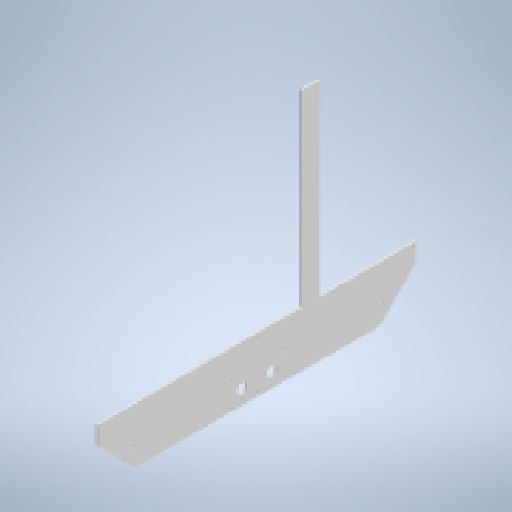
# Autodesk Inventor part: Outside Chassi Plate low
Saved by Autodesk Inventor 2023 (Build 270158000, 158)
## iProperties
Created: 2022-09-05
Part Number: Outside Chassi Plate low
Material: Generic
Document SubType Name: Modeling
Designer: deli
Density: 1 g/cm^3
Appearance: Default
Author: deli
Autodesk Inventor part; units mm, degrees
ref_plane "YZ Plane" through (0, 0, 0) normal (1, 0, 0) x (0, 1, 0)
ref_plane "XZ Plane" through (0, 0, 0) normal (0, 1, 0) x (-1, 0, 0)
ref_plane "XY Plane" through (0, 0, 0) normal (0, 0, 1) x (1, 0, 0)
sketch "Sketch1" plane through (0, 0, 0) normal (1, 0, 0) x (0, 1, 0)
  line L0 (-213.0456, 506.9498) -> (-238.0456, 506.9498)
  line L1 (-238.0456, 506.9498) -> (-289.5596, 456.0589)
  line L2 (-213.0456, 56.9498) -> (-238.0456, 56.9498)
  circle A0 centre (-263.0456, 456.9498) radius 2
  circle A1 centre (-263.0456, 456.9498) radius 48 construction
  arc A2 (-251.1195, 456.4491) -> (-274.9659, 457.5739) centre (-263.0456, 456.9498) ccw construction
  circle A3 centre (-263.0456, 106.9498) radius 48 construction
  arc A4 (-274.9659, 106.3258) -> (-251.1195, 107.4505) centre (-263.0456, 106.9498) ccw construction
  circle A5 centre (-263.0456, 106.9498) radius 2
  circle A6 centre (-270.2956, 303.2411) radius 7
  circle A7 centre (-270.2956, 260.6586) radius 7
  circle A8 centre (-270.2956, 303.2411) radius 18.75 construction
  circle A9 centre (-270.2956, 260.6586) radius 18.75 construction
  arc A10 (-283.0106, 303.9067) -> (-257.5745, 302.707) centre (-270.2956, 303.2411) ccw construction
  arc A11 (-257.5745, 261.1927) -> (-283.0106, 259.9929) centre (-270.2956, 260.6586) ccw construction
  line L3 (-251.1195, 456.4491) -> (-257.5745, 302.707) construction
  line L4 (-283.0106, 303.9067) -> (-274.9659, 457.5739) construction
  line L5 (-257.5745, 261.1927) -> (-251.1195, 107.4505) construction
  line L6 (-274.9659, 106.3258) -> (-283.0106, 259.9929) construction
  circle A12 centre (-255.8131, 281.9498) radius 2
  circle A13 centre (-284.7782, 281.9498) radius 2
  circle A14 centre (-286.0456, 320.3437) radius 2
  circle A15 centre (-286.0456, 243.5559) radius 2
  circle A16 centre (-252.9008, 245.2319) radius 2
  circle A17 centre (-218.0456, 501.9498) radius 2
  circle A18 centre (-218.0456, 61.9498) radius 2
  arc A19 (-291.0456, 229.9036) -> (-291.0456, 229.9036) centre (-268.2956, 229.9036) ccw
  line L7 (-291.0456, 189.1468) -> (-291.0456, 229.9036)
  arc A20 (-291.0456, 189.1468) -> (-291.0456, 189.1468) centre (-268.2956, 189.1468) ccw
  arc A21 (-289.5596, 456.0589) -> (-291.0456, 452.5019) centre (-286.0456, 452.5019) ccw
  line L8 (-291.0456, 452.5019) -> (-291.0456, 229.9036)
  line L9 (-238.0456, 56.9498) -> (-289.5596, 107.8407)
  line L10 (-291.0456, 189.1468) -> (-291.0456, 111.3977)
  circle A22 centre (-252.9008, 318.6677) radius 2
  arc A23 (-291.0456, 111.3977) -> (-289.5596, 107.8407) centre (-286.0456, 111.3977) ccw
  circle A24 centre (-218.0456, 391.9498) radius 2
  circle A25 centre (-218.0456, 281.9498) radius 2
  circle A26 centre (-218.0456, 171.9498) radius 2
  circle A27 centre (-286.0456, 359.8587) radius 2
  circle A28 centre (-286.0456, 399.3738) radius 2
  line L11 (51.9544, 193.3998) -> (-213.0456, 193.3998)
  line L12 (-213.0456, 218.7998) -> (51.9544, 218.7998)
  line L13 (51.9544, 218.7998) -> (51.9544, 193.3998)
  line L14 (-213.0456, 506.9498) -> (-213.0456, 218.7998)
  line L15 (-213.0456, 193.3998) -> (-213.0456, 56.9498)
  line L16 (-197.5778, 237.8081) -> (102.4222, 237.8081) construction
  circle A29 centre (107.0222, 326.3581) radius 5 construction
  line L17 (-197.5778, 237.8081) -> (102.4222, 237.8081) construction
  circle A30 centre (107.0222, 326.3581) radius 5 construction
  circle A31 centre (43.9544, 207.6873) radius 2
  circle A32 centre (-240.0456, 207.6873) radius 2
  point P0 (0, 0)
  dimension "d43" = 450
  dimension "d44" = 4
  dimension "d46" = 96
  dimension "d47" = 23.8732
  dimension "d48" = 96
  dimension "d49" = 4
  dimension "d51" = 23.8732
  dimension "d54" = 50
  dimension "d55" = 50
  dimension "d56" = 25
  dimension "d57" = 25
  dimension "d58" = 14
  dimension "d59" = 14
  dimension "d60" = 37.5
  dimension "d61" = 37.5
  dimension "d62" = 25.4648
  dimension "d63" = 25.4648
  dimension "d64" = 179.407
  dimension "d65" = 179.407
  dimension "d66" = 179.407
  dimension "d67" = 179.407
  dimension "d68" = 153.8776
  dimension "d70" = 153.8776
  dimension "d74" = 4
  dimension "d75" = 4
  dimension "d77" = 4
  dimension "d78" = 4
  dimension "d91" = 5
  dimension "d92" = 5
  dimension "d94" = 2.5
  dimension "d95" = 2.5
  dimension "d97" = 2.5
  dimension "d103" = 4
  dimension "d106" = 4
  dimension "d108" = 5
  dimension "d112" = 5
  dimension "d120" = 4
  dimension "d124" = 28
  dimension "d125" = 20.75
  dimension "d127" = 20.75
  dimension "d142" = 4
  dimension "d143" = 2.5
  dimension "d144" = 4
  dimension "d145" = 4
  dimension "d146" = 18
  dimension "d147" = 18
  dimension "d148" = 5
  dimension "d149" = 5
  dimension "d150" = 440
  dimension "d151" = 4
  dimension "d152" = 4
  dimension "d153" = 4
  dimension "d154" = 4
  dimension "d157" = 5
  dimension "d161" = 110
  dimension "d162" = 110
  dimension "d163" = 110
  dimension "d166" = 5
  dimension "d167" = 5
  dimension "d169" = 4
  dimension "d170" = 5
  dimension "d171" = 12
  dimension "d172" = 79.0301
  dimension "d173" = 39.515
  constraints: 32 end point, 31 centre point, 17 point on circle, 16 tangent, 7 vertical, 6 coincident, 4 perpendicular, 2 concentric, 2 horizontal, 1 parallel
  measures "d43" distance of L0.start L2.start
  measures "d44" diameter of A0
  measures "d46" diameter of A1
  measures "d47" diameter of A2
  measures "d48" diameter of A3
  measures "d49" diameter of A5
  measures "d51" diameter of A4
  measures "d54" distance from line of A0.centre L0
  measures "d55" distance from line of L2 A5.centre
  measures "d56" distance of L0.start L0.end
  measures "d57" distance of L2.start L2.end
  measures "d58" diameter of A6
  measures "d59" diameter of A7
  measures "d60" diameter of A8
  measures "d61" diameter of A9
  measures "d62" diameter of A10
  measures "d63" diameter of A11
  measures "d68" distance of L3.start L3.end
  measures "d70" distance of L5.start L5.end
  measures "d74" diameter of A14
  measures "d75" diameter of A13
  measures "d77" diameter of A12
  measures "d78" diameter of A16
  measures "d103" diameter of A17
  measures "d106" diameter of A18
  measures "d108" distance from line of L0 A17.centre
  measures "d112" distance from line of L2 A18.centre
  measures "d120" diameter of A15
  measures "d124" distance from line of A0.centre L7
  measures "d125" distance from line of L7 A6.centre
  measures "d127" distance from line of L7 A7.centre
  measures "d142" distance from line of L5 A16.centre
  measures "d144" distance from line of L3 A22.centre
  measures "d145" diameter of A22
  measures "d146" distance from line of A0.centre L1
  measures "d147" distance from line of L9 A3.centre
  measures "d148" radius of A21
  measures "d149" radius of A23
  measures "d150" distance of A18.centre A17.centre
  measures "d151" diameter of A24
  measures "d152" diameter of A25
  measures "d153" diameter of A26
  measures "d154" diameter of A27
  measures "d157" distance from line of L8 A27.centre
  measures "d161" distance of A24.centre A17.centre
  measures "d162" distance of A24.centre A25.centre
  measures "d163" distance of A25.centre A26.centre
  measures "d166" distance from line of L8 A14.centre
  measures "d167" distance from line of L10 A15.centre
  measures "d169" diameter of A28
  measures "d170" distance from line of L8 A28.centre
  measures "d172" distance of A28.centre A14.centre
  measures "d173" distance of A27.centre A28.centre
extrude "Extrusion1" add sketch "Sketch1" along normal blind 3.175 contours L14 L12 L13 L11 L15 L2 L9 A23 L10 A20 A19 A16 A15 L8 A21 L1 L0 | A19 A15 A16 A20 | A19 A20 L7 | A20 A19 | A19 A20 | A28 | A31 | A32
body "Solid1"
